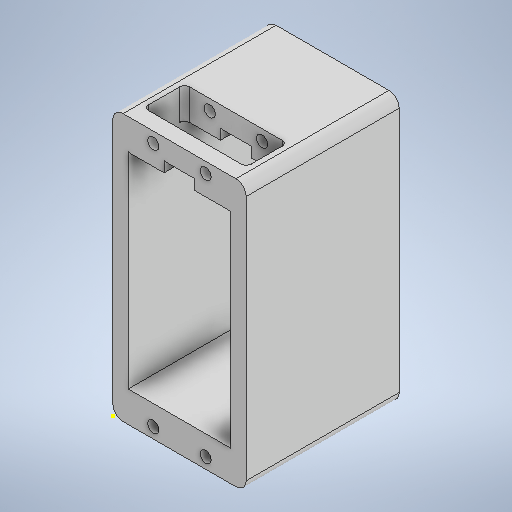
# Autodesk Inventor part: NewServoMount
Saved by Autodesk Inventor 2025.2 (Build 292293000, 293)
## iProperties
Category: <PART CATAGORY>
Created: 2025-01-23
Part Number: NewServoMount
Material: Generic
Document SubType Name: Modeling
Designer: Carriett 4
Density: 1 g/cm^3
Appearance: Default
Title: <TITLE>
Author: Carriett 4
Revision Number: 1
Autodesk Inventor part; units mm, degrees
ref_plane "YZ Plane" through (0, 0, 0) normal (1, 0, 0) x (0, 1, 0)
ref_plane "XZ Plane" through (0, 0, 0) normal (0, 1, 0) x (-1, 0, 0)
ref_plane "XY Plane" through (0, 0, 0) normal (0, 0, 1) x (1, 0, 0)
sketch "Sketch6" plane through (0, 0, 0) normal (0, 0, 1) x (1, 0, 0)
  line L0 (2, 0) -> (24, 0)
  line L1 (24, 52) -> (2, 52)
  line L2 (0, 50) -> (0, 2)
  line L3 (3, 6) -> (23, 6)
  line L4 (23, 6) -> (23, 46)
  line L5 (13, 6) -> (13, 46) construction
  line L6 (16, 46) -> (16, 48)
  line L7 (10, 48) -> (10, 46)
  line L8 (23, 46) -> (16, 46)
  line L9 (10, 46) -> (3, 46)
  arc A0 (2, 52) -> (0, 50) centre (2, 50) ccw
  arc A1 (26, 50) -> (24, 52) centre (24, 50) ccw
  arc A2 (24, 0) -> (26, 2) centre (24, 2) ccw
  arc A3 (0, 2) -> (2, 0) centre (2, 2) ccw
  line L10 (3, 26) -> (23, 26) construction
  line L11 (26, 2) -> (26, 50)
  line L12 (3, 46) -> (3, 6)
  line L13 (10, 48) -> (16, 48)
  point P0 (0, 0)
  dimension "d122" = 52
  dimension "d126" = 6
  dimension "d127" = 6
  dimension "d131" = 3
  dimension "d132" = 2
  dimension "d159" = 13
  dimension "d162" = 10
  dimension "d163" = 10
  dimension "d164" = 3
  dimension "d165" = 3
  dimension "d166" = 20
  dimension "d167" = 40
  constraints: 28 end point, 8 point on circle, 8 tangent, 4 centre point, 4 parallel, 3 equal radius, 3 horizontal, 2 midpoint, 2 point on line, 2 vertical, 1 perpendicular
  measures "d122" distance between parallel lines of L0 L1
  measures "d126" distance between parallel lines of L0 L3
  measures "d127" distance of L7.start L6.end
  measures "d131" distance between parallel lines of L6 L5
  measures "d132" radius of A0
  measures "d159" distance between parallel lines of L5 L2
  measures "d162" distance between parallel lines of L4 L5
  measures "d163" distance between parallel lines of L12 L5
  measures "d164" distance between parallel lines of L2 L12
  measures "d165" distance between parallel lines of L11 L4
  measures "d166" distance between parallel lines of L4 L12
  measures "d167" distance between parallel lines of L8 L3
extrude "Extrusion3" add sketch "Sketch6" against normal blind 29.833
sketch "Sketch7" plane through (0, 0, 0) normal (0, 0, 1) x (1, 0, 0)
  point P0 (0, 0)
sketch "Sketch8" plane through (0, 0, 0) normal (0, 0, 1) x (1, 0, 0)
  circle A0 centre (7.9, 49.9) radius 1.095
  circle A1 centre (18.1, 49.9) radius 1.095
  line L0 (3, 46) -> (10, 46) projected
  line L1 (16, 46) -> (23, 46) projected
  line L2 (10, 48) -> (16, 48) projected
  line L3 (13, 48) -> (13, 6) construction
  line L4 (3, 6) -> (23, 6) projected
  line L5 (5, 6) -> (5, 46) projected
  line L6 (5, 26) -> (23, 26) construction
  line L7 (23, 46) -> (23, 6) projected
  circle A2 centre (7.9, 2.1) radius 1.095
  circle A3 centre (18.1, 2.1) radius 1.095
  point P0 (0, 0)
  dimension "d149" = 2.19
  dimension "d150" = 2.19
  dimension "d151" = 3.9
  dimension "d152" = 3.9
  dimension "d153" = 5.1
  dimension "d154" = 5.1
  constraints: 4 centre point, 4 end point, 3 midpoint, 2 symmetric about line, 4 other
  measures "d149" diameter of A0
  measures "d150" diameter of A1
  measures "d151" distance from line of L0 A0.centre
  measures "d152" distance from line of A1.centre L1
  measures "d153" distance from line of A1.centre L3
  measures "d154" distance from line of A0.centre L3
extrude "Extrusion4" cut sketch "Sketch8" against normal blind 33.25
sketch "Sketch9" plane through (2, 52, 0) normal (0, 1, 0) x (1, 0, 0)
  line L0 (1, 3) -> (21, 3)
  line L1 (21, 3) -> (21, 11)
  line L2 (21, 11) -> (1, 11)
  line L3 (1, 11) -> (1, 3)
  line L4 (22, 0) -> (0, 0) projected
  line L5 (0, 0) -> (0, 29.833) projected
  point P0 (-2, 0)
  dimension "d168" = 20
  dimension "d169" = 8
  dimension "d171" = 3
  dimension "d172" = 1
  constraints: 8 end point, 2 parallel, 1 horizontal, 1 perpendicular
  measures "d168" distance of L2.end L1.end
  measures "d169" distance of L1.end L0.end
  measures "d171" distance between parallel lines of L4 L0
  measures "d172" distance between parallel lines of L5 L3
extrude "Extrusion5" cut sketch "Sketch9" against normal blind 6
fillet "Fillet1" radius 1 1 edges at (23, 49, -11)
fillet "Fillet2" radius 1 3 edges at (23, 49, -3) (3, 49, -11) (3, 49, -3)
body "Solid2"
